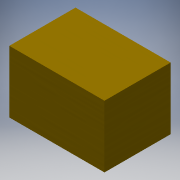
# Autodesk Inventor part: winch
Saved by Autodesk Inventor 2017 (Build 210142000, 142)
## iProperties
Created: 2017-02-22
Part Number: winch
Material: Generic
Document SubType Name: Modeling
Designer: user
Density: 1 g/cm^3
Appearance: Gold
Author: user
Autodesk Inventor part; units mm, degrees
ref_plane "YZ Plane" through (0, 0, 0) normal (1, 0, 0) x (0, 1, 0)
ref_plane "XZ Plane" through (0, 0, 0) normal (0, 1, 0) x (-1, 0, 0)
ref_plane "XY Plane" through (0, 0, 0) normal (0, 0, 1) x (1, 0, 0)
sketch "Sketch1" plane through (0, 0, 0) normal (0, 0, 1) x (1, 0, 0)
  line L0 (-190, -896.7461) -> (-190, -1116.7461) projected
  line L1 (-190, -1116.7461) -> (-710, -1116.7461) projected
  line L2 (-710, -1116.7461) -> (-710, -896.7461) projected
  line L3 (-710, -896.7461) -> (-190, -896.7461) projected
  line L4 (-150, -20) -> (150, -20) projected
  line L5 (150, -20) -> (150, 20) projected
  line L6 (150, 20) -> (-190, 20) projected
  line L7 (-190, 20) -> (-190, -856.7461) projected
  line L8 (-190, -856.7461) -> (-710, -856.7461) projected
  line L9 (-710, -856.7461) -> (-710, 20) projected
  arc A0 (-710, 20) -> (-1028.8395, 243.2539) centre (-947.5818, 20) ccw projected
  line L10 (-1028.8395, 243.2539) -> (-1015.1587, 205.6661) projected
  arc A1 (-750, 20) -> (-1015.1587, 205.6661) centre (-947.5818, 20) ccw projected
  line L11 (-750, 20) -> (-750, -1156.7461) projected
  line L12 (-750, -1156.7461) -> (-150, -1156.7461) projected
  line L13 (-150, -1156.7461) -> (-150, -20) projected
  circle A2 centre (-270, -776.7461) radius 6 projected
  line L14 (-350, -856.7461) -> (-190, -856.7461) projected
  line L15 (-190, -856.7461) -> (-190, -696.7461) projected
  line L16 (-350, -696.7461) -> (-190, -696.7461) projected
  line L17 (-350, -856.7461) -> (-350, -696.7461) projected
  line L18 (-190, -856.7461) -> (-420, -856.7461)
  line L19 (-420, -856.7461) -> (-420, -696.7461)
  line L20 (-420, -696.7461) -> (-190, -696.7461)
  line L21 (-190, -696.7461) -> (-190, -856.7461)
  point P0 (0, 0)
  dimension "d0" = 230
  constraints: 8 end point, 2 parallel, 1 collinear, 1 horizontal, 1 perpendicular
  measures "d0" distance of L19.end L20.end
extrude "Extrusion1" add sketch "Sketch1" against normal blind 150 contours L7 L8 L17 L16 | L17 L8 L19 L20 | A2
body "Solid1"
